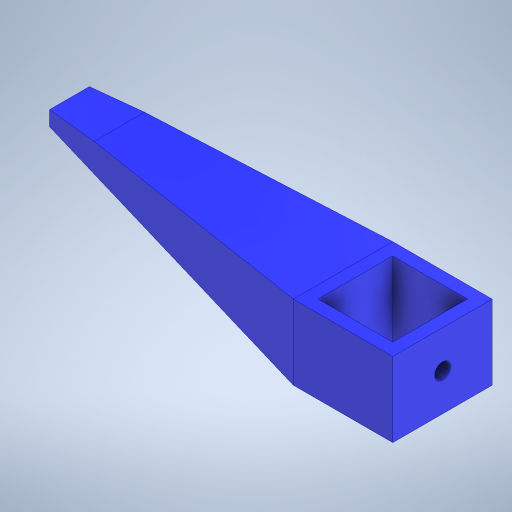
# Autodesk Inventor part: endeff_3dp4
Saved by Autodesk Inventor 2024 (Build 280153000, 153)
## iProperties
Created: 2024-12-14
Part Number: endeff_3dp4
Material: ABS プラスチック
Document SubType Name: Modeling
Designer: hirek
Density: 1.06 g/cm^3
Appearance: 青 - 壁塗料 - 光沢
Author: hirek
Autodesk Inventor part; units mm, degrees
ref_plane "YZ Plane" through (0, 0, 0) normal (1, 0, 0) x (0, 1, 0)
ref_plane "XZ Plane" through (0, 0, 0) normal (0, 1, 0) x (-1, 0, 0)
ref_plane "XY Plane" through (0, 0, 0) normal (0, 0, 1) x (1, 0, 0)
sketch "スケッチ1" plane through (0, 0, 0) normal (0, 1, 0) x (-1, 0, 0)
  line L0 (0, 0) -> (20, 0)
  line L1 (20, 0) -> (20, -20)
  line L2 (20, -20) -> (0, -20)
  line L3 (0, -20) -> (0, 0)
  line L4 (17.5, -2.5) -> (2.5, -2.5)
  line L5 (2.5, -2.5) -> (2.5, -17.5)
  line L6 (2.5, -17.5) -> (17.5, -17.5)
  line L7 (17.5, -17.5) -> (17.5, -2.5)
  dimension "d0" = 20
  dimension "d1" = 20
  dimension "d2" = 15
  dimension "d3" = 15
  dimension "d4" = 2.5
  dimension "d5" = 2.5
  constraints: 16 end point, 4 parallel, 2 horizontal, 2 perpendicular
  measures "d0" distance of L1.end L2.end
  measures "d1" distance of L0.end L1.end
  measures "d2" distance of L6.end L5.end
  measures "d3" distance of L5.end L4.end
  measures "d4" distance between parallel lines of L7 L1
  measures "d5" distance between parallel lines of L4 L0
extrude "押し出し1" add sketch "スケッチ1" along normal blind 15
sketch "スケッチ2" plane through (-20, 0, 0) normal (0, 0, 1) x (1, 0, 0)
  line L0 (20, 0) -> (-55, 0)
  line L1 (-55, 0) -> (-55, 17.5)
  line L2 (-55, 17.5) -> (20, 17.5)
  line L3 (20, 17.5) -> (20, 0)
  line L4 (-55, 17.5) -> (-45, 17.5)
  line L5 (-45, 17.5) -> (-45, 14.5)
  line L6 (-45, 14.5) -> (-55, 14.5)
  line L7 (-55, 14.5) -> (-55, 17.5)
  line L8 (0, 0) -> (0, 15) projected
  line L9 (-55, 14.5) -> (0, 0)
  line L10 (-45, 17.5) -> (0, 15)
  point P0 (-45, 17.5)
  dimension "d8" = 75
  dimension "d9" = 17.5
  dimension "d10" = 10
  dimension "d11" = 3
  constraints: 20 end point, 4 parallel, 2 horizontal, 2 perpendicular
  measures "d8" distance of L1.end L2.end
  measures "d9" distance of L0.end L1.end
  measures "d10" distance of L5.end L6.end
  measures "d11" distance of L4.end L5.end
extrude "押し出し2" add sketch "スケッチ2" against normal blind 20 contours L9 L6 L5 L10 L8 | L1 L2 L5 L6
sketch "スケッチ3" plane through (0, 0, 0) normal (0, -1, 0) x (1, 0, 0)
  line L0 (-75, 0) -> (-75, -20) projected
  line L1 (0, 0) -> (0, -20) projected
  line L2 (-75, -14) -> (0, -14)
  line L3 (0, -14) -> (0, -6)
  line L4 (0, -6) -> (-75, -6)
  line L5 (-75, -6) -> (-75, -14)
  line L6 (-20, -20) -> (-75, -20) projected
  line L7 (-75, -14) -> (-20, -20)
  line L8 (-20, 0) -> (0, 0) projected
  line L9 (-75, -6) -> (-20, 0)
  line L10 (-75, -20) -> (-20, -20)
  line L11 (-20, -20) -> (-20, 0)
  line L12 (-20, 0) -> (-75, 0)
  line L13 (-75, 0) -> (-75, -20)
  dimension "d14" = 8
  dimension "d15" = 6
  constraints: 20 end point, 4 parallel, 2 horizontal, 2 perpendicular, 2 point on line
  measures "d14" distance of L3.end L2.end
  measures "d15" distance between parallel lines of L2 L6
extrude "押し出し3" cut sketch "スケッチ3" against normal through all contours L12 L9 L0 | L7 L6 L0
sketch "スケッチ4" plane through (0, 0, 0) normal (1, 0, 0) x (0, 0, -1)
  line L0 (0, 0) -> (0, 15) projected
  line L1 (0, 7.5) -> (20, 7.5)
  line L2 (20, 0) -> (20, 15) projected
  point P0 (10, 7.5)
  constraints: 3 midpoint, 2 end point
hole "穴1" at (0, 7.5, -10) direction (-1, 0, 0) diameter 3.2 depth 8 tip angle 118
